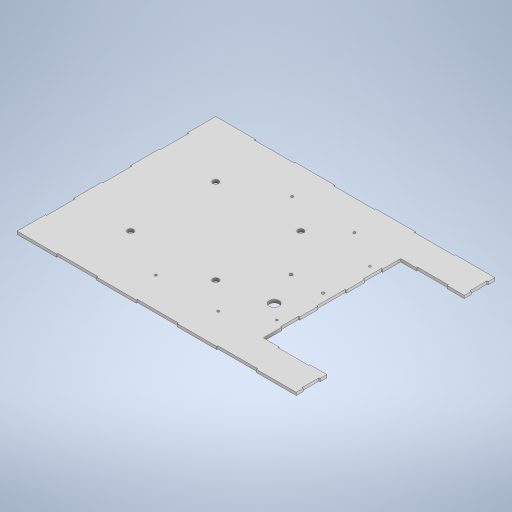
# Autodesk Inventor part: top
Saved by Autodesk Inventor 2023 (Build 270158000, 158)
## iProperties
Created: 2023-04-26
Part Number: top
Material: Generic
Document SubType Name: Modeling
Designer: Unnar
Density: 1 g/cm^3
Appearance: Default
Author: Unnar
Autodesk Inventor part; units mm, degrees
ref_plane "YZ Plane" through (0, 0, 0) normal (1, 0, 0) x (0, 1, 0)
ref_plane "XZ Plane" through (0, 0, 0) normal (0, 1, 0) x (-1, 0, 0)
sketch "Sketch1" plane through (0, 0, 0) normal (0, 1, 0) x (-1, 0, 0)
  line L0 (277.2864, 213.6884) -> (-214.7136, 213.6884)
  line L1 (-214.7136, -136.3116) -> (277.2864, -136.3116)
  line L2 (277.2864, -136.3116) -> (277.2864, 213.6884)
  line L3 (-214.7136, 159.6884) -> (-102.7136, 159.6884)
  line L4 (-102.7136, 159.6884) -> (-102.7136, -82.3116)
  line L5 (-102.7136, -82.3116) -> (-214.7136, -82.3116)
  line L6 (-214.7136, 213.6884) -> (-214.7136, 159.6884)
  line L7 (-214.7136, -82.3116) -> (-214.7136, -136.3116)
  point P0 (0, 0)
  dimension "d0" = 350
  dimension "d1" = 492
  dimension "d2" = 112
  dimension "d3" = 112
  dimension "d4" = 54
  dimension "d5" = 54
  constraints: 16 end point, 4 parallel, 3 perpendicular, 2 horizontal
  measures "d0" distance between parallel lines of L1 L0
  measures "d1" distance of L1.start L1.end
  measures "d2" distance of L4.end L5.end
  measures "d3" distance between parallel lines of L6 L4
  measures "d4" distance of L5.end L1.start
  measures "d5" distance of L0.end L3.start
extrude "Extrusion1" add sketch "Sketch1" along normal blind 5
sketch "Sketch2" plane through (0, 5, 0) normal (0, 1, 0) x (1, 0, 0)
  line L0 (214.7136, 136.3116) -> (-277.2864, 136.3116) projected
  line L1 (-207.2864, 136.3116) -> (-137.2864, 136.3116)
  line L2 (-137.2864, 136.3116) -> (-137.2864, 134.3116)
  line L3 (-137.2864, 134.3116) -> (-207.2864, 134.3116)
  line L4 (-207.2864, 134.3116) -> (-207.2864, 136.3116)
  line L5 (-67.2864, 136.3116) -> (4.7136, 136.3116)
  line L6 (4.7136, 136.3116) -> (4.7136, 134.3116)
  line L7 (4.7136, 134.3116) -> (-67.2864, 134.3116)
  line L8 (-67.2864, 134.3116) -> (-67.2864, 136.3116)
  line L9 (74.7136, 136.3116) -> (144.7136, 136.3116)
  line L10 (144.7136, 136.3116) -> (144.7136, 134.3116)
  line L11 (144.7136, 134.3116) -> (74.7136, 134.3116)
  line L12 (74.7136, 134.3116) -> (74.7136, 136.3116)
  line L13 (-277.2864, -213.6884) -> (214.7136, -213.6884) projected
  line L14 (144.7136, -213.6884) -> (74.7136, -213.6884)
  line L15 (74.7136, -213.6884) -> (74.7136, -211.6884)
  line L16 (74.7136, -211.6884) -> (144.7136, -211.6884)
  line L17 (144.7136, -211.6884) -> (144.7136, -213.6884)
  line L18 (4.7136, -213.6884) -> (-67.2864, -213.6884)
  line L19 (-67.2864, -213.6884) -> (-67.2864, -211.6884)
  line L20 (-67.2864, -211.6884) -> (4.7136, -211.6884)
  line L21 (4.7136, -211.6884) -> (4.7136, -213.6884)
  line L22 (-137.2864, -213.6884) -> (-207.2864, -213.6884)
  line L23 (-207.2864, -213.6884) -> (-207.2864, -211.6884)
  line L24 (-207.2864, -211.6884) -> (-137.2864, -211.6884)
  line L25 (-137.2864, -211.6884) -> (-137.2864, -213.6884)
  line L26 (-277.2864, 136.3116) -> (-277.2864, -213.6884) projected
  line L27 (-277.2864, 86.3116) -> (-275.2864, 86.3116)
  line L28 (-275.2864, 86.3116) -> (-275.2864, 36.3116)
  line L29 (-275.2864, 36.3116) -> (-277.2864, 36.3116)
  line L30 (-277.2864, 36.3116) -> (-277.2864, 86.3116)
  line L31 (-277.2864, -13.6884) -> (-275.2864, -13.6884)
  line L32 (-275.2864, -13.6884) -> (-275.2864, -63.6884)
  line L33 (-275.2864, -63.6884) -> (-277.2864, -63.6884)
  line L34 (-277.2864, -63.6884) -> (-277.2864, -13.6884)
  line L35 (-277.2864, -113.6884) -> (-275.2864, -113.6884)
  line L36 (-275.2864, -113.6884) -> (-275.2864, -163.6884)
  line L37 (-275.2864, -163.6884) -> (-277.2864, -163.6884)
  line L38 (-277.2864, -163.6884) -> (-277.2864, -113.6884)
  line L39 (214.7136, 82.3116) -> (214.7136, 136.3116) projected
  line L40 (214.7136, 124.3116) -> (212.7136, 124.3116)
  line L41 (212.7136, 124.3116) -> (212.7136, 94.3116)
  line L42 (212.7136, 94.3116) -> (214.7136, 94.3116)
  line L43 (214.7136, 94.3116) -> (214.7136, 124.3116)
  line L44 (214.7136, -213.6884) -> (214.7136, -159.6884) projected
  line L45 (214.7136, -171.6884) -> (212.7136, -171.6884)
  line L46 (212.7136, -171.6884) -> (212.7136, -201.6884)
  line L47 (212.7136, -201.6884) -> (214.7136, -201.6884)
  line L48 (214.7136, -201.6884) -> (214.7136, -171.6884)
  line L49 (102.7136, 82.3116) -> (214.7136, 82.3116) projected
  line L50 (214.7136, -159.6884) -> (102.7136, -159.6884) projected
  line L51 (184.7136, 82.3116) -> (130.7136, 82.3116)
  line L52 (130.7136, 82.3116) -> (130.7136, 84.3116)
  line L53 (130.7136, 84.3116) -> (184.7136, 84.3116)
  line L54 (184.7136, 84.3116) -> (184.7136, 82.3116)
  line L55 (184.7136, -159.6884) -> (130.7136, -159.6884)
  line L56 (130.7136, -159.6884) -> (130.7136, -161.6884)
  line L57 (130.7136, -161.6884) -> (184.7136, -161.6884)
  line L58 (184.7136, -161.6884) -> (184.7136, -159.6884)
  line L59 (102.7136, -159.6884) -> (102.7136, 82.3116) projected
  line L60 (102.7136, 50.3116) -> (100.7136, 50.3116)
  line L61 (100.7136, 50.3116) -> (100.7136, 18.3116)
  line L62 (100.7136, 18.3116) -> (102.7136, 18.3116)
  line L63 (102.7136, 18.3116) -> (102.7136, 50.3116)
  line L64 (102.7136, -13.6884) -> (100.7136, -13.6884)
  line L65 (100.7136, -13.6884) -> (100.7136, -63.6884)
  line L66 (100.7136, -63.6884) -> (102.7136, -63.6884)
  line L67 (102.7136, -63.6884) -> (102.7136, -13.6884)
  line L68 (102.7136, -127.6884) -> (100.7136, -127.6884)
  line L69 (100.7136, -127.6884) -> (100.7136, -95.6884)
  line L70 (100.7136, -95.6884) -> (102.7136, -95.6884)
  line L71 (102.7136, -95.6884) -> (102.7136, -127.6884)
  point P0 (0, 0)
  point P1 (-207.2864, -213.6884)
  point P2 (130.7136, -159.6884)
  dimension "d8" = 2
  dimension "d9" = 2
  dimension "d10" = 2
  dimension "d11" = 2
  dimension "d12" = 50
  dimension "d13" = 50
  dimension "d14" = 50
  dimension "d15" = 50
  dimension "d16" = 50
  dimension "d17" = 50
  dimension "d18" = 12
  dimension "d19" = 12
  dimension "d20" = 12
  dimension "d21" = 12
  dimension "d22" = 70
  dimension "d23" = 70
  dimension "d24" = 72
  dimension "d25" = 70
  dimension "d26" = 70
  dimension "d27" = 70
  dimension "d28" = 2
  dimension "d29" = 2
  dimension "d30" = 30
  dimension "d32" = 2
  dimension "d33" = 2
  dimension "d34" = 2
  dimension "d35" = 32
  dimension "d36" = 32
  dimension "d37" = 32
  dimension "d39" = 32
  dimension "d40" = 32
  dimension "d41" = 32
  dimension "d42" = 50
  dimension "d45" = 72
  dimension "d46" = 70
  dimension "d47" = 28
  dimension "d48" = 28
  dimension "d49" = 54
  dimension "d50" = 54
  dimension "d51" = 30
  constraints: 128 end point, 32 parallel, 31 point on line, 16 horizontal, 16 perpendicular
  measures "d8" distance between parallel lines of L0 L3
  measures "d9" distance between parallel lines of L26 L28
  measures "d10" distance between parallel lines of L13 L24
  measures "d11" distance between parallel lines of L39 L41
  measures "d12" distance between parallel lines of L27 L0
  measures "d13" distance of L27.end L28.end
  measures "d14" distance of L31.end L32.end
  measures "d15" distance of L35.end L36.end
  measures "d16" distance between parallel lines of L29 L31
  measures "d17" distance between parallel lines of L35 L33
  measures "d18" distance between parallel lines of L0 L40
  measures "d19" distance between parallel lines of L49 L42
  measures "d20" distance between parallel lines of L50 L45
  measures "d21" distance between parallel lines of L13 L47
  measures "d22" distance between parallel lines of L39 L10
  measures "d23" distance of L10.end L11.end
  measures "d24" distance of L6.end L7.end
  measures "d25" distance between parallel lines of L6 L12
  measures "d26" distance between parallel lines of L2 L8
  measures "d27" distance of L2.end L3.end
  measures "d28" distance between parallel lines of L50 L57
  measures "d29" distance between parallel lines of L49 L53
  measures "d30" distance between parallel lines of L39 L54
  measures "d32" distance between parallel lines of L59 L61
  measures "d33" distance between parallel lines of L59 L65
  measures "d34" distance between parallel lines of L59 L69
  measures "d35" distance from line of L49.start L60
  measures "d36" distance of L60.end L61.end
  measures "d37" distance between parallel lines of L64 L62
  measures "d39" distance between parallel lines of L70 L66
  measures "d40" distance of L68.end L69.end
  measures "d41" distance between parallel lines of L50 L68
  measures "d42" distance of L66.end L64.start
  measures "d45" distance of L19.end L20.end
  measures "d46" distance between parallel lines of L26 L4
  measures "d47" distance between parallel lines of L59 L52
  measures "d48" distance between parallel lines of L59 L56
  measures "d49" distance of L56.end L57.end
  measures "d50" distance of L52.end L53.end
  measures "d51" distance between parallel lines of L44 L58
extrude "Extrusion2" cut sketch "Sketch2" against normal blind 10 contours L10 L11 L12 L0 | L39 L42 L41 L40 | L6 L7 L8 L0 | L49 L52 L53 L54 | L2 L3 L4 L0 | L59 L62 L61 L60 | L27 L28 L29 L26 | L59 L66 L65 L64 | L31 L32 L33 L26 | L59 L68 L69 L70 | L35 L36 L37 L26 | L50 L58 L57 L56 | L23 L24 L25 L13 | L19 L20 L21 L13 | L44 L47 L46 L45 | L15 L16 L17 L13
sketch "Sketch3" plane through (0, 5, 0) normal (0, 1, 0) x (1, 0, 0)
  circle A0 centre (-177.2864, 36.3116) radius 5
  line L0 (-277.2864, 136.3116) -> (-277.2864, 86.3116) projected
  line L1 (-207.2864, 136.3116) -> (-277.2864, 136.3116) projected
  point P0 (0, 0)
  dimension "d52" = 100
  dimension "d53" = 100
  dimension "d54" = 10
  constraints: 1 centre point
  measures "d52" distance from line of L0 A0.centre
  measures "d53" distance from line of L1 A0.centre
  measures "d54" diameter of A0
extrude "Extrusion3" cut sketch "Sketch3" against normal blind 10
pattern_linear "Rectangular Pattern1" count 2 spacing 150 along (0, 0, 1) count 2 spacing 150 along (1, 0, 0) of "Extrusion3"
sketch "Sketch5" plane through (0, 5, 0) normal (0, 1, 0) x (1, 0, 0)
  circle A0 centre (87.1836, 43.3116) radius 1.9
  circle A1 centre (22.1836, 81.3116) radius 1.9
  circle A2 centre (-87.8164, 81.3116) radius 1.9
  line L0 (102.7136, 50.3116) -> (102.7136, 82.3116) projected
  line L1 (102.7136, -13.6884) -> (102.7136, 18.3116) projected
  line L2 (-67.2864, 136.3116) -> (-137.2864, 136.3116) projected
  line L3 (74.7136, 136.3116) -> (4.7136, 136.3116) projected
  point P0 (0, 0)
  dimension "d63" = 15.53
  dimension "d64" = 3.8
  dimension "d65" = 80.53
  dimension "d66" = 3.8
  dimension "d67" = 3.8
  dimension "d68" = 190.53
  dimension "d69" = 55
  dimension "d70" = 55
  dimension "d71" = 93
  constraints: 3 centre point
  measures "d63" distance from line of L0 A0.centre
  measures "d64" diameter of A0
  measures "d65" distance from line of L0 A1.centre
  measures "d66" diameter of A1
  measures "d67" diameter of A2
  measures "d68" distance from line of L1 A2.centre
  measures "d69" distance from line of L2 A2.centre
  measures "d70" distance from line of L3 A1.centre
  measures "d71" distance from line of L3 A0.centre
extrude "Extrusion4" cut sketch "Sketch5" against normal blind 10
sketch "Sketch6" plane through (0, 5, 0) normal (0, 1, 0) x (1, 0, 0)
  line L0 (100.7136, -63.6884) -> (100.7136, -13.6884) projected
  line L1 (100.7136, -38.6884) -> (-275.2864, -38.6884)
  line L2 (-275.2864, -63.6884) -> (-275.2864, -13.6884) projected
  point P0 (0, 0)
  constraints: 2 end point, 2 midpoint
ref_plane "Work Plane2" through (100.7136, 5, 38.6884) normal (0, 0, 1) x (1, 0, 0)
mirror "Mirror1" about plane through (100.7136, 5, 38.6884) normal (0, 0, 1) of "Extrusion4"
sketch "Sketch8" plane through (0, 5, 0) normal (0, 1, 0) x (1, 0, 0)
  circle A0 centre (86.9636, -38.6884) radius 2.5
  circle A1 centre (30.4636, -38.6884) radius 2.5
  line L0 (130.7136, -159.6884) -> (102.7136, -159.6884) projected
  line L1 (102.7136, -95.6884) -> (102.7136, -63.6884) projected
  point P0 (0, 0)
  point P1 (116.7136, -159.6884)
  dimension "d78" = 5
  dimension "d79" = 121
  dimension "d80" = 121
  dimension "d81" = 15.75
  dimension "d82" = 56.5
  dimension "d83" = 5
  constraints: 2 centre point, 1 midpoint
  measures "d78" diameter of A1
  measures "d79" vertical distance of point (116.714, -159.688) A0.centre
  measures "d80" distance from line of L0 A1.centre
  measures "d81" distance from line of L1 A0.centre
  measures "d82" distance of A0.centre A1.centre
  measures "d83" diameter of A0
extrude "Extrusion5" cut sketch "Sketch8" against normal blind 10
sketch "Sketch9" plane through (0, 5, 0) normal (0, 1, 0) x (1, 0, 0)
  circle A0 centre (59.7136, -97.6884) radius 8.5
  line L0 (4.7136, -213.6884) -> (74.7136, -213.6884) projected
  line L1 (102.7136, -95.6884) -> (102.7136, -63.6884) projected
  point P0 (0, 0)
  dimension "d86" = 17
  dimension "d87" = 116
  dimension "d88" = 43
  constraints: 1 centre point
  measures "d86" diameter of A0
  measures "d87" distance from line of L0 A0.centre
  measures "d88" distance from line of L1 A0.centre
extrude "Extrusion6" cut sketch "Sketch9" against normal blind 10
body "Solid1"
